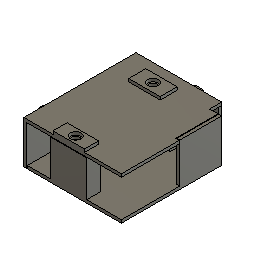
tail box (Autodesk Fusion 360 design; units mm, degrees)
part number: 2026-04-21-21-24-14-663
Autodesk Fusion 360 part; units mm, degrees
note: some values were not read from the file. Chosen so that the rebuilt part matches the saved one: which face or edge a step refers to; where a step starts.
sketch "front side" plane through (0, 0, 0) normal (0, 0, 1) x (1, 0, 0)
  line L0 (-1, 0) -> (-31.6, 0)
  line L1 (-31.6, 0) -> (-31.6, 12.3)
  line L2 (-31.6, 12.3) -> (-1, 12.3)
  line L3 (-1, 12.3) -> (-1, 0)
  line L4 (-32.6, 13.3) -> (0, 13.3)
  line L5 (0, 13.3) -> (0, 12.3)
  line L6 (0, 12.3) -> (-32.6, 12.3)
  line L7 (-32.6, 12.3) -> (-32.6, 13.3)
  line L8 (-1, 12.3) -> (0, 12.3)
  line L9 (0, 12.3) -> (0, 0)
  line L10 (0, 0) -> (-1, 0)
  line L11 (-1, 0) -> (-1, 12.3)
  line L12 (0, -1) -> (-32.6, -1)
  line L13 (-32.6, -1) -> (-32.6, 0)
  line L14 (-32.6, 0) -> (0, 0)
  line L15 (0, 0) -> (0, -1)
  line L16 (-31.6, 0) -> (-32.6, 0)
  line L17 (-32.6, 0) -> (-32.6, 12.3)
  line L18 (-32.6, 12.3) -> (-31.6, 12.3)
  line L19 (-31.6, 12.3) -> (-31.6, 0)
  circle A0 centre (-16.3, 5.65) radius 3.75
  circle A1 centre (-16.3, 5.65) radius 2.75
  circle A2 centre (-16.3, 5.65) radius 1.25
  circle A3 centre (-16.3, 5.65) radius 1.75
  line L20 (-31.6, 0) -> (-28.6, 0)
  line L21 (-28.6, 0) -> (-28.6, 12.3)
  line L22 (-28.6, 0) -> (-28.6, 0.1849)
  line L23 (-28.6, 0) -> (-23.6, 0)
  line L24 (-23.6, 0) -> (-23.6, 12.3)
  line L25 (-28.6, 0) -> (-11.6, 0)
  line L26 (-11.6, 0) -> (-11.6, 12.3)
  line L27 (-1, 0) -> (-4, 0)
  line L28 (-4, 0) -> (-4, 12.3)
  line L29 (-1, 0) -> (-1, -1)
  line L30 (-31.6, 0) -> (-31.6, -1)
  line L31 (-1, 12.3) -> (-1, 13.3)
  dimension "d10" = 7.5
  dimension "d11" = 5.5
  dimension "d12" = 2.5
  dimension "d13" = 3.5
  dimension "d14" = 3
  dimension "d15" = 5
  dimension "d16" = 17
  dimension "d38" = 3
  constraint horizontal L0
  constraint vertical L1
  constraint horizontal L2
  constraint vertical L3
  constraint horizontal L4
  constraint vertical L5
  constraint horizontal L6
  constraint vertical L7
  constraint horizontal L8
  constraint vertical L9
  constraint horizontal L10
  constraint vertical L11
  constraint horizontal L12
  constraint vertical L13
  constraint horizontal L14
  constraint vertical L15
  constraint horizontal L16
  constraint vertical L17
  constraint horizontal L18
  constraint vertical L19
  constraint concentric A0 A1
  constraint concentric A0 A2
  constraint concentric A0 A3
  constraint coincident L0 L20.end
  constraint coincident L6 L21.end
  constraint coincident L21 L22.end
  constraint coincident L14 L23.end
  constraint coincident L6 L24.end
  constraint coincident L0 L25.end
  constraint coincident L2 L26.end
  constraint coincident L0 L27.end
  constraint coincident L6 L28.end
  constraint coincident L12 L29.end
  constraint perpendicular L12 L29
  constraint coincident L12 L30.end
  constraint perpendicular L12 L30
  constraint coincident L4 L31.end
  constraint perpendicular L4 L31
  measures "d10" diameter of A0
  measures "d11" diameter of A1
  measures "d12" diameter of A2
  measures "d13" diameter of A3
  measures "d14" distance of L0.end L20.end
  measures "d15" distance of L20.end L23.end
  measures "d16" distance of L20.end L25.end
  measures "d38" distance of L0.start L27.end
extrude "Extrude1" add sketch "front side" against normal blind 36.6 contours L0 L12 L14 L20 L23 L25 L27 L29 L30 | L10 L12 L14 L15 L29 | L12 L13 L14 L16 L30 | L1 L6 L14 L16 L17 L18 L19 makes body 1
extrude "Extrude2" add sketch "front side" against normal blind 4.7 contours L0 L2 L6 L14 L24 L25 L26 | A0 | A1 | A2 | A3 bodies 1
extrude "Extrude3" add sketch "front side" against normal blind 4.7 from surface at -27.8 contours L0 L2 L6 L14 L24 L25 L26 | L0 L2 L6 L14 L21 L22 L23 L24 L25 | A0 | A1 | A2 | A3 bodies 1
extrude "Extrude4" add sketch "front side" against normal blind 1 from surface at -32.5 contours L0 L2 L3 L6 L11 L14 L27 L28 | L0 L2 L6 L14 L26 L28 | L0 L2 L6 L14 L24 L25 L26 | L0 L2 L6 L14 L21 L22 L23 L24 L25 | A0 | A1 | A2 | A3 bodies 1
extrude "Extrude5" cut 1 faces at (-21.4, -0.6667, -36.6) along direction (0, 0, 1) blind 0.1 on bodies 1 bodies 1
extrude "Extrude6" add sketch "front side" along normal blind 17 from surface at -36.5 contours L3 L6 L8 L9 L10 L11 L14 bodies 1
extrude "Extrude7" add sketch "front side" against normal blind 1 from surface at -36.5 separate body contours L0 L2 L3 L6 L11 L14 L27 L28 | L3 L6 L8 L9 L10 L11 L14 | L0 L2 L6 L14 L26 L28 | L0 L2 L6 L14 L24 L25 L26 | L0 L2 L6 L14 L21 L22 L23 L24 L25 | L0 L1 L2 L6 L14 L19 L20 L21 L22 | L1 L6 L14 L16 L17 L18 L19 | A0 | A1 | A2 | A3 makes body 3
extrude "Extrude8" add sketch "front side" along normal blind 1 from surface at -37.5 contours L0 L12 L14 L20 L23 L25 L27 L29 L30 | L10 L12 L14 L15 L29 | L12 L13 L14 L16 L30 bodies 3
extrude "Extrude9" cut sketch "front side" along normal blind 1 from surface at -37.5 contours L0 L2 L3 L6 L11 L14 L27 L28 bodies 3
extrude "Extrude10" add sketch "front side" along normal up to surface (37.5 mm away) from surface at -37.5 contours L4 L5 L6 L8 L31 | L2 L4 L6 L7 L18 L31 bodies 3
extrude "Extrude11" cut sketch "front side" along normal blind 1 from surface at -37.5 contours A2 | A3 bodies 3
extrude "Extrude12" add sketch "front side" against normal blind 1 from surface at -37.5 contours A0 | A1 | A3 bodies 3
extrude "Extrude13" add sketch "front side" against normal blind 2.5 from surface at -38.5 contours A0 bodies 3
extrude "Extrude14" cut 1 faces at (-12.2, 12.3, -12.1667) along direction (0, -1, 0) blind 0.2 on bodies 3 bodies 1
extrude "Extrude15" cut 1 faces at (-27.75, 5.65, -36.5) along direction (0, 0, 1) blind 0.2 on bodies 3 bodies 1
sketch "top side" plane through (0, 0, 0) normal (0, 1, 0) x (1, 0, 0)
  line L0 (-14.85, 27.8, 13.3) -> (-25.35, 27.8, 13.3)
  line L1 (-25.35, 27.8, 13.3) -> (-25.35, 33.5, 13.3)
  line L2 (-25.35, 33.5, 13.3) -> (-14.85, 33.5, 13.3)
  line L3 (-14.85, 33.5, 13.3) -> (-14.85, 27.8, 13.3)
  line L4 (-12.35, 4.7, 13.3) -> (-22.85, 4.7, 13.3)
  line L5 (-22.85, 4.7, 13.3) -> (-22.85, 0, 13.3)
  line L6 (-22.85, 0, 13.3) -> (-12.35, 0, 13.3)
  line L7 (-12.35, 0, 13.3) -> (-12.35, 4.7, 13.3)
  circle A0 through (-15.85, 2.35, 13.3) (-18.475, 3.8655, 13.3) (-18.475, 0.8345, 13.3)
  circle A1 through (-16.35, 2.35, 13.3) (-18.225, 3.4325, 13.3) (-18.225, 1.2675, 13.3)
  circle A2 through (-16.8, 2.35, 13.3) (-18, 3.0428, 13.3) (-18, 1.6572, 13.3)
  circle A3 through (-18.35, 30.65, 13.3) (-20.975, 32.1655, 13.3) (-20.975, 29.1345, 13.3)
  circle A4 through (-18.85, 30.65, 13.3) (-20.725, 31.7325, 13.3) (-20.725, 29.5675, 13.3)
  circle A5 through (-19.3, 30.65, 13.3) (-20.5, 31.3428, 13.3) (-20.5, 29.9572, 13.3)
  circle A6 through (-17.85, 30.65, 13.3) (-21.225, 32.5986, 13.3) (-21.225, 28.7014, 13.3)
  circle A7 through (-15.35, 2.35, 13.3) (-18.725, 4.2986, 13.3) (-18.725, 0.4014, 13.3)
  line L8 (-1, 33.5, 13.3) -> (-4, 33.5, 13.3)
  line L9 (-4, 33.5, 13.3) -> (-4, 38.5, 13.3)
  line L10 (-4, 38.5, 13.3) -> (-1, 38.5, 13.3)
  line L11 (-1, 38.5, 13.3) -> (-1, 33.5, 13.3)
  dimension "d58" = 3.5
  dimension "d59" = 2.5
  dimension "d60" = 1.6
  dimension "d61" = 3.5
  dimension "d62" = 2.5
  dimension "d63" = 1.6
  dimension "d64" = 4.5
  dimension "d65" = 4.5
  dimension "d96" = 5
sketch "top side (curves 13.3 mm off its plane)" plane through (0, 13.3, 0) normal (0, 1, 0) x (1, 0, 0)
  line L0 (-14.85, 27.8) -> (-25.35, 27.8)
  line L1 (-25.35, 27.8) -> (-25.35, 33.5)
  line L2 (-25.35, 33.5) -> (-14.85, 33.5)
  line L3 (-14.85, 33.5) -> (-14.85, 27.8)
  line L4 (-12.35, 4.7) -> (-22.85, 4.7)
  line L5 (-22.85, 4.7) -> (-22.85, 0)
  line L6 (-22.85, 0) -> (-12.35, 0)
  line L7 (-12.35, 0) -> (-12.35, 4.7)
  circle A0 centre (-17.6, 2.35) radius 1.75
  circle A1 centre (-17.6, 2.35) radius 1.25
  circle A2 centre (-17.6, 2.35) radius 0.8
  circle A3 centre (-20.1, 30.65) radius 1.75
  circle A4 centre (-20.1, 30.65) radius 1.25
  circle A5 centre (-20.1, 30.65) radius 0.8
  circle A6 centre (-20.1, 30.65) radius 2.25
  circle A7 centre (-17.6, 2.35) radius 2.25
  line L8 (-1, 33.5) -> (-4, 33.5)
  line L9 (-4, 33.5) -> (-4, 38.5)
  line L10 (-4, 38.5) -> (-1, 38.5)
  line L11 (-1, 38.5) -> (-1, 33.5)
extrude "Extrude16" add sketch "top side (curves 13.3 mm off its plane)" along normal blind 1 contours A6 | A7 bodies 3
extrude "Extrude17" cut sketch "top side (curves 13.3 mm off its plane)" against normal blind 1 contours A1 | A2 | A4 | A5 bodies 3
extrude "Extrude18" cut sketch "top side (curves 13.3 mm off its plane)" against normal blind 3.5 from surface at -1.2 contours A2 | A5 bodies 1
extrude "Extrude19" add 1 faces at (-28.4167, 5.9833, -37.5) along direction (0, 0, -1) blind 1 on bodies 3 bodies 3
extrude "Extrude20" cut 1 faces at (-0.6667, 8.0667, -19.5) along direction (0, 0, -1) blind 16.8 on bodies 1 bodies 1
extrude "Extrude21" cut 1 faces at (-31.6, 4.0333, -12.1) along direction (-1, 0, 0) blind 1 on bodies 1 bodies 1
extrude "Extrude22" cut sketch "front side" along normal through all from surface at -36.3 contours L10 L12 L14 L15 L29 | L12 L13 L14 L16 L30 bodies 1
extrude "Extrude23" add sketch "front side" along normal up to surface (36.5 mm away) from surface at -36.5 contours L12 L13 L14 L16 L30 | L1 L6 L14 L16 L17 L18 L19 bodies 3
extrude "Extrude24" add sketch "front side" along normal blind 17 from surface at -36.5 contours L3 L6 L8 L9 L10 L11 L14 | L10 L12 L14 L15 L29 bodies 3
extrude "Extrude25" add sketch "front side" along normal up to near side of body 3 contours L10 L12 L14 L15 L29 bodies 1
extrude "Extrude26" cut 1 faces at (-1, -0.6667, -29.4333) along direction (-1, 0, 0) blind 0.2 on bodies 1 bodies 1
extrude "Extrude27" cut 1 faces at (-0.7333, -0.3333, -19.5) along direction (0, 0, 1) blind 0.2 on bodies 1 bodies 1
extrude "Extrude28" cut 1 faces at (-31.6, -0.3333, -24.2) along direction (1, 0, 0) blind 0.2 on bodies 1 bodies 1
extrude "Extrude29" cut sketch "top side (curves 13.3 mm off its plane)" against normal up to surface (14.3 mm away) from surface at 0 contours L8 L9 L10 L11 bodies 1 3
extrude "Extrude30" cut 1 faces at (-0.3333, 4.1, -38.5) along direction (0, 0, 1) blind 19.2 on bodies 3 bodies 3
extrude "Extrude31" add 1 faces at (-0.7333, -0.3333, -19.3) along direction (0, 0, -1) blind 0.2 on bodies 1 bodies 1
extrude "Extrude32" add sketch "front side" against normal up to surface (14 mm away) from surface at -19.5 contours L3 L6 L8 L9 L10 L11 L14 | L10 L12 L14 L15 L29 | L4 L5 L6 L8 L31 bodies 1
extrude "Extrude33" add 1 faces at (-1.2, -0.6667, -28.5) along direction (1, 0, 0) blind 0.2 on bodies 1 bodies 1
extrude "Extrude34" cut 1 faces at (-1, 12.6333, -24.0333) along direction (-1, 0, 0) blind 0.2 on bodies 3 bodies 3
extrude "Extrude35" cut 1 faces at (-28.4167, 5.9833, -38.5) along direction (0, 0, 1) blind 1 on bodies 3 bodies 3
extrude "Extrude36" add 1 faces at (-12.9075, 5.3271, -41) along direction (0, 0, -1) blind 1 on bodies 3 bodies 3
extrude "Extrude37" add 1 faces at (-14.0649, 5.4513, -38.5) along direction (0, 0, -1) blind 1 on bodies 3 bodies 3
extrude "Extrude38" cut 1 faces at (-14.7278, 5.501, -37.5) along direction (0, 0, -1) blind 1 on bodies 3 bodies 3
extrude "Extrude39" add sketch "top side (curves 13.3 mm off its plane)" along normal blind 1 contours L0 L1 L2 L3 | L4 L5 L6 L7 bodies 3
sketch "Sketch4" plane through (0, 0, 0) normal (1, 0, 0) x (0, 0, -1)
  line L0 (0, -1) -> (0, 13.3)
  line L1 (0, 6.15) -> (10.6, 6.15)
  circle A0 centre (10.6, 6.15) radius 2.5
  dimension "d122" = 10.6
  dimension "d124" = 5
  constraint vertical L0
  constraint midpoint L0 L1.start
  constraint perpendicular L0 L1
  measures "d122" distance of L1.start L1.end
  measures "d124" diameter of A0
extrude "Extrude40" add sketch "Sketch4" against normal blind 5 from surface at -32.6 bodies 3
named bodies: "body", "head"
